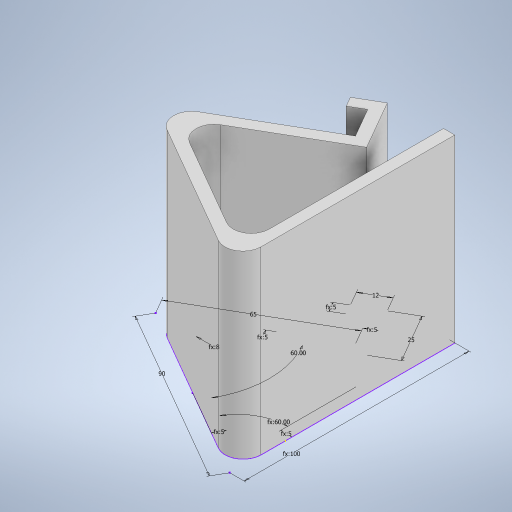
# Autodesk Inventor part: phonestand2DSketch_afterExtrusion
Saved by Autodesk Inventor 2024.2 (Build 282272000, 272)
## iProperties
Created: 2025-02-05
Part Number: phonestand2DSketch_afterExtrusion
Material: Generic
Document SubType Name: Modeling
Designer: veillettem
Density: 1 g/cm^3
Appearance: Default
Author: veillettem
Autodesk Inventor part; units mm, degrees
ref_plane "YZ Plane" through (0, 0, 0) normal (1, 0, 0) x (0, 1, 0)
ref_plane "XZ Plane" through (0, 0, 0) normal (0, 1, 0) x (-1, 0, 0)
ref_plane "XY Plane" through (0, 0, 0) normal (0, 0, 1) x (1, 0, 0)
sketch "PhoneStandProfile" plane through (0, 0, 0) normal (0, 1, 0) x (-1, 0, 0)
  line L0 (5, -75.5038) -> (0, -75.5038)
  line L1 (0, -75.5038) -> (0, 10.6398)
  line L2 (12, 17.568) -> (65.9423, -13.5756)
  line L3 (65.9423, -27.432) -> (21.6506, -53.0038)
  line L4 (29.1506, -65.9942) -> (35.2128, -62.4942)
  line L5 (37.7128, -66.8243) -> (27.3205, -72.8243)
  line L6 (27.3205, -72.8243) -> (14.8205, -51.1737)
  line L7 (14.8205, -51.1737) -> (55.9423, -27.432)
  line L8 (55.9423, -13.5756) -> (17, 8.9077)
  line L9 (5, 1.9795) -> (5, -75.5038)
  line L10 (21.6506, -53.0038) -> (29.1506, -65.9942)
  line L11 (35.2128, -62.4942) -> (37.7128, -66.8243)
  arc A0 (55.9423, -27.432) -> (55.9423, -13.5756) centre (51.9423, -20.5038) ccw
  arc A1 (65.9423, -27.432) -> (65.9423, -13.5756) centre (61.9423, -20.5038) ccw
  arc A2 (17, 8.9077) -> (5, 1.9795) centre (13, 1.9795) ccw
  arc A3 (12, 17.568) -> (0, 10.6398) centre (8, 10.6398) ccw
  point P0 (0, 0)
  point P1 (0, 24.4962)
  point P2 (77.9423, -20.5038)
  point P3 (38.2819, -18.3391)
  point P4 (5, -36.7621)
  point P5 (38.9711, 1.9962)
  point P6 (43.7965, -40.2179)
  point P7 (21.0705, -61.999)
  point P8 (2.5, -75.5038)
  dimension "internalAngle" = 60
  dimension "d1" = 60
  dimension "d2" = 5
  dimension "d3" = 5
  dimension "d4" = 5
  dimension "d7" = 5
  dimension "d8" = 5
  dimension "d9" = 25
  dimension "d10" = 100
  dimension "d11" = 90
  dimension "d12" = 65
  dimension "d13" = 12
  constraints: 24 end point, 8 point on circle, 8 tangent, 5 midpoint, 4 centre point, 4 parallel, 4 point on line, 3 equal radius, 3 perpendicular, 2 vertical, 1 other
  measures "internalAngle" angle of L7 L8
  measures "d1" angle of L9 L8
  measures "d2" distance from line of L1 point (5, -36.762)
  measures "d3" distance from line of L8 point (38.971, 1.996)
  measures "d4" distance from line of point (43.796, -40.218) L7
  measures "d7" distance between parallel lines of L5 L4
  measures "d8" distance between parallel lines of L6 L10
  measures "d9" distance between parallel lines of L5 L7
  measures "d10" vertical distance of point (0, 24.496) point (2.5, -75.504)
  measures "d11" distance of point (0, 24.496) point (77.942, -20.504)
  measures "d12" distance of point (77.942, -20.504) L3.end
  measures "d13" distance of L5.start L5.end
extrude "MainBody" add sketch "PhoneStandProfile" along normal blind 80
sketch "Rectangle" plane through (-37.7128, 0, -66.8243) normal (-0.5, 0, -0.8660254) x (-0.8660254, 0, 0.5)
  line L0 (-12, 0) -> (-12, 80) projected
  line L1 (0.2233, 48) -> (-12, 48)
  line L2 (-12, 48) -> (-12, 32)
  line L3 (-12, 32) -> (0.2233, 32)
  line L4 (0.2233, 32) -> (0.2233, 48)
  line L5 (-12, 0) -> (0, 0) projected
  line L6 (-12, 80) -> (0, 80) projected
  point P0 (0.7519, 0)
  point P1 (-6, 80)
  point P2 (-5.8884, 48)
  point P3 (-12, 48)
  dimension "distanceFromRightEdge" = 32
  dimension "distanceFromLeftEdge" = 32
  constraints: 8 end point, 2 midpoint, 2 parallel, 1 horizontal, 1 perpendicular, 1 point on line
  measures "distanceFromRightEdge" distance between parallel lines of L5 L3
  measures "distanceFromLeftEdge" vertical distance of point (-6, 80) point (-5.888, 48)
extrude "CentralNotch" cut sketch "Rectangle" against normal up to surface (20 mm away)
equation "\"d1\" = internalAngle"
equation "\"d2\" = thickness"
equation "\"d3\" = thickness"
equation "\"d4\" = thickness"
equation "\"d7\" = thickness"
equation "\"d8\" = thickness"
equation "\"d10\" = baseLength"
equation "\"d15\" = width"
equation "\"distanceFromLeftEdge\" = distanceFromRightEdge"
equation "\"d19\" = width"
equation "\"thickness\" = 5"
equation "\"baseLength\" = 100"
equation "\"width\" = 80"
equation "\"filletRadius_1\" = 8"
body "Solid1"
